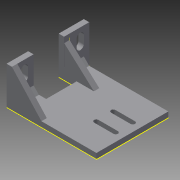
# Autodesk Inventor part: bart z endstop bracket plain switch v1
Saved by Autodesk Inventor 2014 SP1 (Build 180222100, 222)
## iProperties
Created: 2015-07-08
Part Number: bart z endstop bracket plain switch v1
Material: Generic
Document SubType Name: Modeling
Designer: Mon
Density: 1 g/cm^3
Appearance: Default
Author: Mon
Autodesk Inventor part; units mm, degrees
ref_plane "YZ Plane" through (0, 0, 0) normal (1, 0, 0) x (0, 1, 0)
ref_plane "XZ Plane" through (0, 0, 0) normal (0, 1, 0) x (-1, 0, 0)
ref_plane "XY Plane" through (0, 0, 0) normal (0, 0, 1) x (1, 0, 0)
sketch "Sketch1" plane through (0, 0, 0) normal (0, 0, 1) x (1, 0, 0)
  line L0 (0, 0) -> (50, 0)
  line L1 (50, 0) -> (50, -40)
  line L2 (50, -40) -> (0, -40)
  line L3 (0, -40) -> (0, 0)
  dimension "d0" = 50
  dimension "d1" = 40
  constraints: 8 end point, 2 parallel, 1 horizontal, 1 perpendicular
  measures "d0" distance of L1.end L2.end
  measures "d1" distance of L0.end L1.end
extrude "Extrusion1" add sketch "Sketch1" along normal blind 3
sketch "Sketch2" plane through (0, 0, 3) normal (0, 0, 1) x (1, 0, 0)
  line L0 (0, -40) -> (50, -40) projected
  line L1 (0, 0) -> (3, 0)
  line L2 (3, 0) -> (3, -40)
  line L3 (3, -40) -> (0, -40)
  line L4 (0, -40) -> (0, 0)
  dimension "d4" = 3
  constraints: 8 end point, 2 parallel, 1 horizontal, 1 perpendicular, 1 point on line
  measures "d4" distance of L2.end L3.end
extrude "Extrusion2" add sketch "Sketch2" along normal blind 18
sketch "Sketch3" plane through (0, 0, 0) normal (0, 1, 0) x (1, 0, 0)
  line L0 (0, 0) -> (3, 0)
  line L1 (3, 0) -> (3, -21)
  line L2 (3, -21) -> (0, -21)
  line L3 (0, -21) -> (0, 0)
  constraints: 8 end point, 2 parallel, 1 horizontal, 1 perpendicular
extrude "Extrusion3" add sketch "Sketch3" along normal blind 3
sketch "Sketch4" plane through (0, 0, 0) normal (0, 0, -1) x (-1, 0, 0)
  line L0 (0, -40) -> (0, 3) projected
  line L1 (-3, 0) -> (-3, 3) projected
  line L2 (-3, 0) -> (-3, -11)
  line L3 (0, -11) -> (-10, -11)
  line L4 (-10, -11) -> (-10, -27.9486)
  line L5 (-10, -27.9486) -> (0, -27.9486)
  point P0 (0, 0)
  dimension "d9" = 11
  dimension "d10" = 10
  constraints: 8 end point, 2 perpendicular, 2 point on line, 1 collinear, 1 parallel
  measures "d9" distance of L1.start L2.end
  measures "d10" distance of L3.start L3.end
extrude "Extrusion4" cut sketch "Sketch4" against normal blind 8
sketch "Sketch6" plane through (0, -40, 0) normal (-1, 0, 0) x (0, 0, 1)
  line L0 (0, 29) -> (8, 29) projected
  line L1 (12, 38) -> (16.5475, 38) construction
  line L2 (12, 36) -> (16.5475, 36)
  line L3 (16.5475, 40) -> (12, 40)
  arc A0 (12, 40) -> (12, 36) centre (12, 38) ccw
  arc A1 (16.5475, 36) -> (16.5475, 40) centre (16.5475, 38) ccw
  point P0 (0, 40)
  point P1 (14.2738, 38)
  constraints: 8 end point, 4 point on circle, 4 tangent, 2 centre point, 2 parallel, 1 midpoint
extrude "Extrusion6" cut sketch "Sketch6" against normal through all
sketch "Sketch7" plane through (0, -40, 0) normal (-1, 0, 0) x (0, 0, 1)
  line L0 (16.5475, 36) -> (12, 36) projected
  line L1 (12, 7) -> (16.5475, 7) construction
  line L2 (12, 5) -> (16.5475, 5)
  line L3 (16.5475, 9) -> (12, 9)
  arc A0 (12, 9) -> (12, 5) centre (12, 7) ccw
  arc A1 (16.5475, 5) -> (16.5475, 9) centre (16.5475, 7) ccw
  point P0 (0, 40)
  point P1 (14.2738, 7)
  dimension "d67" = 4
  constraints: 8 end point, 4 point on circle, 4 tangent, 2 centre point, 2 parallel, 1 midpoint
  measures "d67" diameter of A1
extrude "Extrusion7" cut sketch "Sketch7" against normal through all
sketch "Sketch8" plane through (0, 0, 0) normal (0, 0, -1) x (-1, 0, 0)
  line L0 (0, -27.9486) -> (-10, -27.9486) projected
  line L1 (-57.8737, -20) -> (-13.9473, -20) construction
  line L2 (-46.7188, -20) -> (-46.7188, -15.25) construction
  line L3 (-46.7188, -15.25) -> (-19.9847, -15.25) construction
  line L4 (-19.9847, -15.25) -> (-19.9847, -24.75) construction
  line L5 (-19.9847, -24.75) -> (-61.1977, -24.75) construction
  line L6 (-46.7188, -15.25) -> (-33.3518, -15.25) construction
  line L7 (-45.4688, -16.5) -> (-34.6018, -16.5)
  line L8 (-34.6018, -14) -> (-45.4688, -14)
  arc A0 (-45.4688, -14) -> (-45.4688, -16.5) centre (-45.4688, -15.25) ccw
  arc A1 (-34.6018, -16.5) -> (-34.6018, -14) centre (-34.6018, -15.25) ccw
  line L9 (-46.7188, -20) -> (-46.7188, -24.9647) construction
  arc A2 (-33.3518, -15.25) -> (-33.4221, -15.7265) centre (-33.3518, -15.4935) ccw construction
  line L10 (-33.4221, -15.7265) -> (-33.4221, -27.1874) construction
  line L11 (-46.7188, -24.75) -> (-33.4221, -24.75) construction
  line L12 (-45.4688, -26) -> (-34.6721, -26)
  line L13 (-34.6721, -23.5) -> (-45.4688, -23.5)
  arc A3 (-45.4688, -23.5) -> (-45.4688, -26) centre (-45.4688, -24.75) ccw
  arc A4 (-34.6721, -26) -> (-34.6721, -23.5) centre (-34.6721, -24.75) ccw
  point P0 (0, 0)
  point P1 (-40.0353, -15.25)
  point P2 (-40.0705, -24.75)
  dimension "d71" = 4.75
  dimension "d72" = 9.5
  dimension "d73" = 2.5
  dimension "d76" = 2.5
  constraints: 30 end point, 14 point on circle, 9 point on line, 9 tangent, 6 parallel, 5 centre point, 3 midpoint, 3 perpendicular
  measures "d71" distance of L2.start L2.end
  measures "d72" distance of L3.end L4.end
  measures "d73" diameter of A1
  measures "d76" diameter of A4
chamfer "Chamfer1" distance 3 angle 45 1 edges at (3, -33.9743, 3)
chamfer "Chamfer2" distance 3 angle 45 1 edges at (3, -5.5, 3)
sketch "Sketch11" plane through (0, 0, 0) normal (0, 0, -1) x (-1, 0, 0)
  line L0 (-48.6932, -22.9665) -> (-25.0226, -22.9665) construction
  line L1 (-45, -22.9665) -> (-37, -22.9665) construction
  line L2 (-10, -11) -> (0, -11) projected
  line L3 (0, -11) -> (0, 3) projected
  line L4 (-3, 3) -> (0, 3) projected
  line L5 (-3, 0) -> (-3, 3) projected
  line L6 (-3, 0) -> (-50, 0) projected
  line L7 (-50, 0) -> (-50, -40) projected
  line L8 (-50, -40) -> (0, -40) projected
  line L9 (0, -40) -> (0, -27.9486) projected
  line L10 (0, -27.9486) -> (-10, -27.9486) projected
  line L11 (-10, -27.9486) -> (-10, -11) projected
  point P0 (0, 0)
  point P1 (-41, -22.9665)
  constraints: 4 end point, 1 midpoint
ref_plane "Work Plane1" through (0, -8, 0) normal (0, 1, 0) x (1, 0, 0)
sketch "Sketch14" plane through (0, -8, 0) normal (0, 1, 0) x (1, 0, 0)
  line L0 (3.0794, -17.957) -> (19.7008, -2.8939)
  line L1 (19.7008, -2.8939) -> (3.0794, -2.8939)
  line L2 (3.0794, -2.8939) -> (3.0794, -17.957)
  point P0 (0, 0)
  constraints: 6 end point, 1 horizontal, 1 perpendicular
extrude "Extrusion14" add sketch "Sketch14" against normal blind 3
sketch "Sketch15" plane through (0, -40, 21) normal (0, -1, 0) x (1, 0, 0)
  line L0 (6, -18) -> (50, -18) projected
  line L1 (3, -15) -> (6, -18) projected
  line L2 (3, -15) -> (3, 0) projected
  line L3 (3, 0) -> (19.3977, -18)
  line L4 (3, -15.75) -> (3, 0)
  constraints: 4 end point, 1 collinear, 1 point on line
extrude "Extrusion15" add sketch "Sketch15" against normal blind 3
sketch "Sketch16" plane through (3, 0, 0) normal (1, 0, 0) x (0, 0, -1)
  line L0 (-21, -37) -> (-21, 3) projected
  line L1 (-21, -11) -> (-8, -11)
  line L2 (-8, -11) -> (-8, -27.9486)
  line L3 (-8, -27.9486) -> (-21, -27.9486)
  line L4 (-21, -27.9486) -> (-21, -11)
  constraints: 8 end point, 2 parallel, 1 horizontal, 1 perpendicular, 1 point on line
extrude "Extrusion16" cut sketch "Sketch16" against normal through all
extrude "Extrusion17" cut sketch "Sketch8" against normal through all contours A0 L8 A1 L7
extrude "Extrusion18" cut sketch "Sketch8" against normal through all contours A3 L13 A4 L12
body "Solid1"
